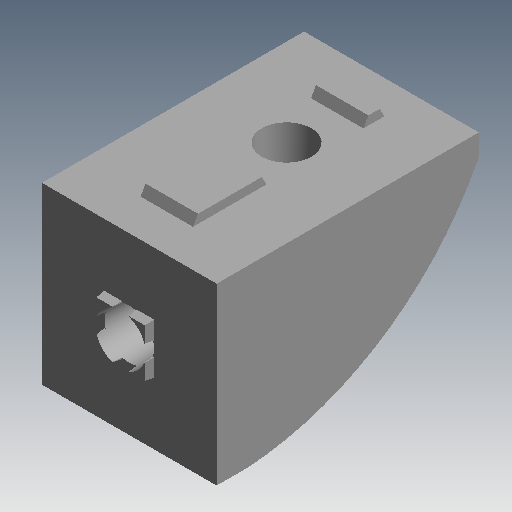
# Autodesk Inventor part: HBLFSNF5-SEC_b
Saved by Autodesk Inventor 2020 (Build 240168000, 168)
## iProperties
Part Number: HBLFSNF5-SEC_b
Material: Generic
Catalog Web Link: www.cadenas.de
Description: HBLFSNF5_brackets-Tabbed Brackets - 1 Slots - HFS5 Series (Aluminum Extrusions 20, 25, 40 Square) - Reversal Tabbed Brackets (Depth 20mm)
Vendor: MISUMI
Document SubType Name: Modeling
Designer: partserver
Manufacturer: MISUMI
Mass: 5.04277 g
Surface Area: 35.0741 cm^2
Volume: 5.04277 cm^3
Density: 1 g/cm^3
Appearance: PSOLRGB-192-192-192
Category: PARTsolutions
Company: MISUMI
PSOL_IDENT_0: {$CADENAS_DATA\23d-libs\misumi\metric\38_al_extrusions_blackets\5\hblfsnf5\hblfsnf5_blacket.prj},186
PSOL_IDENT_1: {VTYP=3D},{NB=HBLFSNF5-SEC_b},{LINA=HBLFSNF5-SEC},{NN=HBLFSNF5_brackets},{DATE=30.03.2018 06:53:34}
PSOL_IDENT_2: ,{GEOMDATE=18.03.2016 03:16:59},{VERSION=},{LINEID=10},{WBVAR=ALT1,ALT2},{WBNUMERIC=}  {NB=HBLFSNF5-
PSOL_IDENT_3: SEC_b},{LINA=HBLFSNF5-SEC},{KT=DUMMY},{PN=HBLFSNF5-SEC},{TYPE=HBLFSNF5},{AS=HCBST5-12},{ASQ=2},{ATN=
PSOL_IDENT_4: HNTT5-5},{ATNQ=2},{ALT1=},{ALT2=-SEC},{ALT2ALG= '' , 'w/o Applicable Screws and Nuts Set' , '-SET' ,
PSOL_IDENT_5: 'with SET (Applicable Screws and Nuts Set)' , '-SST' , 'with SST (Applicable Screws and Nuts Set(St
PSOL_IDENT_6: ainless Steel))' , '-SEU' , 'with SEU (Applicable Screws and Nuts Set(Pre-Assembly Insertion Spring
PSOL_IDENT_7: Nuts))' , '-SSU' , 'with SSU (Applicable Screws and Nuts Set(Pre-Assembly Insertion Spring Nuts Stai
PSOL_IDENT_8: nless Steel))'  , '-SEP' , 'with SEP (Applicable Screws and Nuts Set(Post-Assembly Insertion Spring
PSOL_IDENT_9: Nuts))' , '-SSP' , 'with SSP (Applicable Screws and Nuts Set(Post-Assembly Insertion Spring Nuts Sta
PSOL_IDENT_10: inless Steel))', '-SEC' , 'with SEC (Applicable Screws and Nuts Set(Washer Integrated Screws and Nut
PSOL_IDENT_11: s))' },{SMAT=1010 Carbon Steel Equivalent},{SALT2=3},{NALT2=1},{M=5}
NB: HBLFSNF5-SEC_b
NN: HBLFSNF5_brackets
NT: Tabbed Brackets - 1 Slots - HFS5 Series (Aluminum Extrusions 20, 25, 40 Square) - Reversal Tabbed Brackets (Depth 20mm)
NBSYN: $PN._b
LINA: HBLFSNF5-SEC
CATALOG: Misumi
PN: HBLFSNF5-SEC
TYPE: HBLFSNF5
AS: HCBST5-12
ASQ: 2
ATN: HNTT5-5
ATNQ: 2
ALT1: w/o C (Mounting Holes for Cover)
ALT2: with SEC (Applicable Screws and Nuts Set(Washer Integrated Screws and Nuts))
SUPPLIER: MISUMI
ARTICLENO: HBLFSNF5-SEC_b
BOMINFO: HBLFSNF5-SEC
CREATOR: CADENAS GmbH
Title: HBLFSNF5-SEC
Author: Cadenas PARTsolutions
Comments: Tabbed Brackets - 1 Slots - HFS5 Series (Aluminum Extrusions 20, 25, 40 Square) - Reversal Tabbed Brackets (Depth 20mm)
Autodesk Inventor part; units mm, degrees
sketch "Sketch_1" plane through (0, 0, 0) normal (1, 0, 0) x (0, 0, -1)
  line L0 (-20, 3.4921) -> (-20, 0)
  line L1 (-20, 0) -> (0, 0)
  line L2 (0, 0) -> (0, 30)
  line L3 (0, 30) -> (-2.2048, 30)
  arc A0 (-2.2048, 30) -> (-2.6607, 29.89) centre (-2.2048, 29) ccw
  arc A1 (-2.6607, 29.89) -> (-19.9977, 3.5593) centre (11.93, 1.41) ccw
  arc A2 (-19.9977, 3.5593) -> (-20, 3.4921) centre (-19, 3.4921) ccw
  constraints: 8 end point, 6 point on circle, 3 centre point
extrude "Extrusion1" add sketch "Sketch_1" along normal blind 20
sketch "Sketch_2" plane through (10, 0, 0) normal (1, 0, 0) x (0, 0, -1)
  line L0 (-20, 30) -> (-20, 4.5)
  line L1 (-20, 4.5) -> (-4.5, 4.5)
  line L2 (-4.5, 4.5) -> (-3.1636, 30)
  line L3 (-3.1636, 30) -> (-20, 30)
  constraints: 8 end point
extrude "Extrusion2" cut sketch "Sketch_2" along normal mid plane 15
sketch "Sketch_5" plane through (10, 0, 0) normal (1, 0, 0) x (0, 0, -1)
  line L0 (-0.5, 26.5) -> (-0.5, 23.5)
  line L1 (-0.5, 23.5) -> (1, 24.366)
  line L2 (1, 24.366) -> (1, 25.634)
  line L3 (1, 25.634) -> (-0.5, 26.5)
  constraints: 8 end point
extrude "Extrusion3" add sketch "Sketch_5" along normal mid plane 6
sketch "Sketch_6" plane through (10, 0, 0) normal (1, 0, 0) x (0, 0, -1)
  line L0 (-0.5, 13) -> (-0.5, 4)
  line L1 (-0.5, 4) -> (1, 4.866)
  line L2 (1, 4.866) -> (1, 12.134)
  line L3 (1, 12.134) -> (-0.5, 13)
  constraints: 8 end point
extrude "Extrusion4" add sketch "Sketch_6" along normal mid plane 6
sketch "Sketch_3" plane through (0, 0, 4.5) normal (0, 0, 1) x (1, 0, 0)
  line L0 (3.4955, 4.5) -> (16.5045, 4.5)
  line L1 (16.5045, 4.5) -> (14.4534, 18.6457)
  arc A0 (14.4534, 18.6457) -> (5.5466, 18.6457) centre (10, 18) ccw
  line L2 (5.5466, 18.6457) -> (3.4955, 4.5)
  constraints: 6 end point, 2 point on circle, 1 centre point
extrude "Extrusion5" add sketch "Sketch_3" against normal blind 2 draft 45
sketch "Sketch_7" plane through (0, 0.5, 0) normal (0, 1, 0) x (1, 0, 0)
  line L0 (7.075, -12.925) -> (12.925, -12.925)
  line L1 (12.925, -12.925) -> (12.925, -7.075)
  line L2 (12.925, -7.075) -> (7.075, -7.075)
  line L3 (7.075, -7.075) -> (7.075, -12.925)
  constraints: 8 end point
extrude "Extrusion6" add sketch "Sketch_7" against normal blind 1.5 draft -6
sketch "Sketch_9" plane through (0, 0, 0) normal (0, 1, 0) x (1, 0, 0)
  line L0 (7.075, -10.835) -> (9.165, -10.835)
  line L1 (9.165, -10.835) -> (9.165, -12.925)
  line L2 (9.165, -12.925) -> (10.835, -12.925)
  line L3 (10.835, -12.925) -> (10.835, -10.835)
  line L4 (10.835, -10.835) -> (12.925, -10.835)
  line L5 (12.925, -10.835) -> (12.925, -9.165)
  line L6 (12.925, -9.165) -> (10.835, -9.165)
  line L7 (10.835, -9.165) -> (10.835, -7.075)
  line L8 (10.835, -7.075) -> (9.165, -7.075)
  line L9 (9.165, -7.075) -> (9.165, -9.165)
  line L10 (9.165, -9.165) -> (7.075, -9.165)
  line L11 (7.075, -9.165) -> (7.075, -10.835)
  constraints: 24 end point
extrude "Extrusion7" cut sketch "Sketch_9" against normal blind 1 draft 6
sketch "Sketch_4" plane through (10, 0, 0) normal (1, 0, 0) x (0, 0, -1)
  line L0 (0, 18) -> (-4.5, 18)
  line L1 (-4.5, 18) -> (-4.5, 20.6)
  line L2 (-4.5, 20.6) -> (0, 20.8358)
  line L3 (0, 20.8358) -> (0, 18)
  line L4 (0, 18) -> (-4.5, 18)
  constraints: 10 end point
revolve "Revolution1" cut sketch "Sketch_4" angle 360 about axis through (10, 18, 0) along (0, 0, -1)
sketch "Sketch_8" plane through (10, 0, 0) normal (1, 0, 0) x (0, 0, -1)
  line L0 (-10, -1) -> (-10, 4.5)
  line L1 (-10, 4.5) -> (-7.4, 4.5)
  line L2 (-7.4, 4.5) -> (-7.1118, -1)
  line L3 (-7.1118, -1) -> (-10, -1)
  line L4 (-10, -1) -> (-10, 4.5)
  constraints: 10 end point
revolve "Revolution2" cut sketch "Sketch_8" angle 360 about axis through (10, -1, 10) along (0, -1, 0)
ref_plane "to_bolt1_XY" through (10, 18, 4.5) normal (0, 0, 1) x (1, 0, 0)
ref_plane "to_bolt1_YZ" through (10, 18, 4.5) normal (1, 0, 0) x (0, 1, 0)
ref_plane "to_bolt1_ZX" through (10, 18, 4.5) normal (0, 1, 0) x (0, 0, 1)
ref_plane "to_bolt2_XY" through (10, 4.5, 10) normal (0, 1, 0) x (1, 0, 0)
ref_plane "to_bolt2_YZ" through (10, 4.5, 10) normal (1, 0, 0) x (0, 0, -1)
ref_plane "to_bolt2_ZX" through (10, 4.5, 10) normal (0, 0, -1) x (0, 1, 0)
ref_plane "to_nut1_XY" through (10, 18, -1) normal (0, 0, -1) x (0, 1, 0)
ref_plane "to_nut1_YZ" through (10, 18, -1) normal (0, 1, 0) x (1, 0, 0)
ref_plane "to_nut1_ZX" through (10, 18, -1) normal (1, 0, 0) x (0, 0, -1)
ref_plane "to_nut2_XY" through (10, -1, 10) normal (0, -1, 0) x (0, 0, -1)
ref_plane "to_nut2_YZ" through (10, -1, 10) normal (0, 0, -1) x (1, 0, 0)
ref_plane "to_nut2_ZX" through (10, -1, 10) normal (1, 0, 0) x (0, -1, 0)
body "Solid1"
